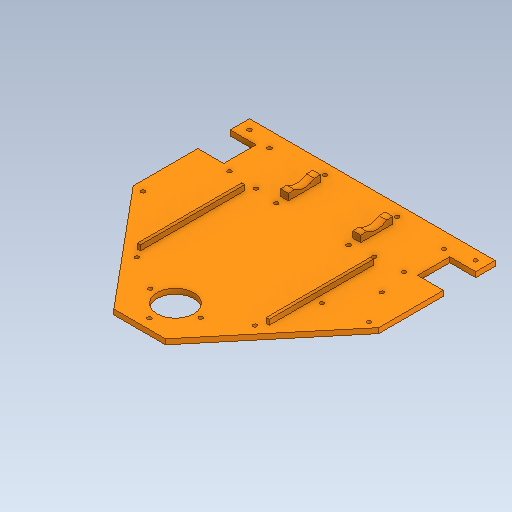
# Autodesk Inventor part: bp_v2
Saved by Autodesk Inventor 2020.3 (Build 243373000, 373)
## iProperties
Created: 2020-06-30
Part Number: bp_v2
Material: PET Plastic
Document SubType Name: Modeling
Designer: Devin
Density: 1.541 g/cm^3
Appearance: Orange
Author: Devin
Autodesk Inventor part; units mm, degrees
ref_plane "YZ Plane" through (0, 0, 0) normal (1, 0, 0) x (0, 1, 0)
ref_plane "XZ Plane" through (0, 0, 0) normal (0, 1, 0) x (-1, 0, 0)
ref_plane "XY Plane" through (0, 0, 0) normal (0, 0, 1) x (1, 0, 0)
sketch "Sketch1" plane through (0, 0, 0) normal (0, 1, 0) x (-1, 0, 0)
  line L0 (0, 0) -> (-190, 0)
  line L1 (0, 0) -> (0, 15)
  line L2 (-170, 15) -> (-170, 40)
  line L3 (-20, 40) -> (-20, 15)
  line L4 (-20, 15) -> (0, 15)
  line L5 (-20, 40) -> (0, 40)
  line L6 (-170, 15) -> (-190, 15)
  line L7 (-170, 40) -> (-190, 40)
  line L8 (0, 15) -> (0, 0)
  line L9 (-190, 0) -> (-190, 15)
  line L10 (-95, 0) -> (-95, 180)
  line L11 (0, 40) -> (0, 90)
  line L12 (-190, 40) -> (-190, 90)
  line L13 (-95, 180) -> (-75, 180)
  line L14 (-75, 180) -> (0, 90)
  line L15 (-95, 180) -> (-115, 180)
  line L16 (-115, 180) -> (-190, 90)
  dimension "d1" = 190
  dimension "d37" = 180
  dimension "d38" = 50
  dimension "d39" = 20
  dimension "d40" = 20
  constraints: 34 end point, 4 horizontal, 4 perpendicular, 3 vertical, 2 parallel, 1 midpoint
  measures "d1" distance of L0.start L0.end
  measures "d37" distance of L10.start L10.end
  measures "d38" distance of L7.end L12.end
  measures "d39" distance of L10.end L13.end
  measures "d40" distance of L10.end L15.end
extrude "Extrusion1" add sketch "Sketch1" along normal blind 4
sketch "Sketch5" plane through (0, 4, 0) normal (0, 1, 0) x (1, 0, 0)
  circle A0 centre (27.5, -12) radius 1.55 projected
  circle A1 centre (27.5, -43) radius 1.55 projected
  circle A2 centre (162.5, -43) radius 1.55 projected
  circle A3 centre (162.5, -12) radius 1.55 projected
  point P0 (0, 0)
extrude "Extrusion2" cut sketch "Sketch5" against normal blind 10
sketch "Sketch6" plane through (0, 4, 0) normal (0, 1, 0) x (1, 0, 0)
  line L0 (20, -15) -> (20, -40) projected
  line L1 (70, -15) -> (70, -40)
  line L2 (70, -40) -> (64, -40)
  line L3 (64, -40) -> (64, -15)
  line L4 (64, -15) -> (70, -15)
  line L5 (190, 0) -> (0, 0) projected
  line L6 (120, -15) -> (120, -40)
  line L7 (120, -40) -> (126, -40)
  line L8 (126, -40) -> (126, -15)
  line L9 (126, -15) -> (120, -15)
  dimension "d24" = 6
  constraints: 16 end point, 2 parallel, 1 perpendicular
  measures "d24" distance of L1.end L2.end
extrude "Extrusion3" add sketch "Sketch6" along normal blind 5
sketch "Sketch7" plane through (126, 4, 40) normal (1, 0, 0) x (0, 0, -1)
  line L0 (0, 0) -> (25, 0) projected
  arc A0 (4.8685, 5) -> (20.1315, 5) centre (12.5, 14.9) ccw
  line L1 (0, 5) -> (25, 5) projected
  line L2 (4.8685, 5) -> (20.1315, 5)
  point P0 (40, -4)
  point P1 (4.8685, 5)
  constraints: 2 end point, 2 point on circle, 1 centre point, 1 collinear, 1 point on line
extrude "Extrusion4" cut sketch "Sketch7" against normal blind 10
sketch "Sketch8" plane through (70, 4, 40) normal (1, 0, 0) x (0, 0, -1)
  line L0 (0, 0) -> (25, 0) projected
  arc A0 (4.8685, 5) -> (20.1315, 5) centre (12.5, 14.9) ccw
  line L1 (25, 5) -> (0, 5) projected
  arc A1 (4.8685, 5) -> (20.1315, 5) centre (12.5, 14.9) ccw projected
  line L2 (20.1315, 5) -> (4.8685, 5)
  point P0 (40, -4)
  point P1 (4.8685, 5)
  constraints: 2 end point, 2 point on circle, 1 centre point, 1 horizontal, 1 point on line
extrude "Extrusion5" cut sketch "Sketch8" against normal blind 10
sketch "Sketch9" plane through (0, 4, 0) normal (0, 1, 0) x (1, 0, 0)
  circle A0 centre (67, -46.379) radius 1.55 projected
  circle A1 centre (123, -46.379) radius 1.55 projected
  circle A2 centre (123, -8.621) radius 1.55 projected
  circle A3 centre (67, -8.621) radius 1.55 projected
  point P0 (0, 0)
extrude "Extrusion6" cut sketch "Sketch9" against normal blind 10
sketch "Sketch10" plane through (0, 4, 0) normal (0, 1, 0) x (1, 0, 0)
  circle A0 centre (67, -46.379) radius 1.55 projected
  circle A1 centre (123, -46.379) radius 1.55 projected
  line L0 (46.35, -50) -> (43.95, -50)
  line L1 (43.95, -50) -> (43.95, -130.85)
  line L2 (43.95, -130.85) -> (46.35, -130.85)
  line L3 (46.35, -130.85) -> (46.35, -50)
  line L4 (146.05, -50) -> (143.65, -50)
  line L5 (143.65, -50) -> (143.65, -130.85)
  line L6 (143.65, -130.85) -> (146.05, -130.85)
  line L7 (146.05, -130.85) -> (146.05, -50)
  point P0 (0, 0)
  dimension "d89" = 2.4
  dimension "d90" = 80.85
  dimension "d92" = 2.4
  dimension "d93" = 80.85
  dimension "d94" = 97.3
  constraints: 16 end point, 4 parallel, 2 horizontal, 2 perpendicular
  measures "d89" distance of L0.start L0.end
  measures "d90" distance of L1.end L0.end
  measures "d92" distance of L4.start L4.end
  measures "d93" distance of L5.end L4.end
  measures "d94" distance between parallel lines of L5 L3
extrude "Extrusion7" add sketch "Sketch10" along normal blind 4 contours L3 L2 L1 L0 | L7 L6 L5 L4
sketch "Sketch14" plane through (0, 4, 0) normal (0, 1, 0) x (1, 0, 0)
  line L0 (190, 0) -> (0, 0) projected
  line L1 (0, 0) -> (0, -7.5)
  line L2 (0, 0) -> (0, -15) projected
  line L3 (0, -90) -> (75, -180) projected
  circle A0 centre (7.5, -7.5) radius 1.55
  circle A1 centre (7.5, -90) radius 1.55
  line L4 (75, -180) -> (115, -180) projected
  circle A2 centre (182.5, -7.5) radius 1.55
  circle A3 centre (182.5, -90) radius 1.55
  circle A4 centre (95, -172.5) radius 1.55
  dimension "d68" = 7.5
  dimension "d71" = 3.1
  dimension "d72" = 3.1
  dimension "d74" = 3.1
  constraints: 5 centre point, 2 end point, 1 midpoint
  measures "d68" distance of L0.end L1.end
  measures "d71" diameter of A0
  measures "d72" diameter of A1
  measures "d74" diameter of A4
extrude "Extrusion10" cut sketch "Sketch14" against normal blind 10
sketch "Sketch15" plane through (0, 4, 0) normal (0, 1, 0) x (1, 0, 0)
  circle A0 centre (140.65, -44.3) radius 1.55 projected
  circle A1 centre (140.65, -136.55) radius 1.55 projected
  circle A2 centre (49.35, -136.55) radius 1.55 projected
  circle A3 centre (49.35, -44.3) radius 1.55 projected
  point P0 (0, 0)
extrude "Extrusion11" cut sketch "Sketch15" against normal blind 10
sketch "Sketch16" plane through (0, 4, 0) normal (0, 1, 0) x (1, 0, 0)
  circle A0 centre (167.6524, -65.2346) radius 1.5 projected
  circle A1 centre (151.6574, -95.6346) radius 1.5 projected
  point P0 (0, 0)
extrude "Extrusion12" cut sketch "Sketch16" against normal blind 10
sketch "Sketch17" plane through (0, 4, 0) normal (0, 1, 0) x (1, 0, 0)
  circle A0 centre (95, -152.3364) radius 14.25
  line L0 (75, -180) -> (115, -180) projected
  point P0 (0, 0)
  dimension "d101" = 28.5
  dimension "d112" = 27.6636
  constraints: 1 centre point
  measures "d101" diameter of A0
  measures "d112" distance from line of L0 A0.centre
extrude "Extrusion13" cut sketch "Sketch17" against normal through all
sketch "Sketch19" plane through (0, 4, 0) normal (0, 1, 0) x (1, 0, 0)
  circle A0 centre (95, -152.3364) radius 14.25 projected
  circle A1 centre (114.5, -152.3364) radius 1.55
  circle A2 centre (75.5, -152.3364) radius 1.55
  point P0 (0, 0)
  dimension "d108" = 3.1
  dimension "d109" = 3.1
  constraints: 2 centre point
  measures "d108" diameter of A1
  measures "d109" diameter of A2
extrude "Extrusion14" cut sketch "Sketch19" against normal blind 5 contours A1 | A2
body "Solid1"
